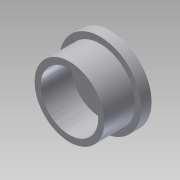
# Autodesk Inventor part: Bouchon PVC
Saved by Autodesk Inventor 2016 (Build 200138000, 138)
## iProperties
Created: 2016-01-27
Part Number: Bouchon PVC
Material: PVC, non plastifié
Document SubType Name: Modeling
Designer: sd
Mass: 14.2475 g
Surface Area: 61.3475 cm^2
Volume: 10.1768 cm^3
Density: 1.4 g/cm^3
Appearance: Lisse - Blanc
Author: sd
Autodesk Inventor part; units mm, degrees
ref_plane "YZ Plane" through (0, 0, 0) normal (1, 0, 0) x (0, 1, 0)
ref_plane "XZ Plane" through (0, 0, 0) normal (0, 1, 0) x (-1, 0, 0)
ref_plane "XY Plane" through (0, 0, 0) normal (0, 0, 1) x (1, 0, 0)
sketch "Esquisse1" plane through (0, 0, 0) normal (0, 1, 0) x (-1, 0, 0)
  circle A0 centre (0, 0) radius 20
  dimension "d0" = 40
  constraints: 1 centre point, 1 coincident
  measures "d0" diameter of A0
extrude "Extrusion1" add sketch "Esquisse1" along normal blind 20
sketch "Esquisse2" plane through (0, 0, 0) normal (0, -1, 0) x (1, 0, 0)
  circle A0 centre (0, 0) radius 20 projected
  circle A1 centre (0, 0) radius 17
  dimension "d3" = 3
  constraints: 1 centre point, 1 coincident
  measures "d3" radial gap between concentric circles of A0 A1
extrude "Extrusion2" cut sketch "Esquisse2" against normal blind 15
sketch "Esquisse3" plane through (0, 0, 0) normal (0, -1, 0) x (1, 0, 0)
  circle A0 centre (0, 0) radius 17 projected
  circle A1 centre (0, 0) radius 14
  dimension "d6" = 3
  constraints: 1 centre point, 1 coincident
  measures "d6" radial gap between concentric circles of A0 A1
extrude "Extrusion3" cut sketch "Esquisse3" against normal blind 15 contours A1
sketch "Esquisse4" plane through (0, 15, 0) normal (0, -1, 0) x (1, 0, 0)
  circle A0 centre (0, 0) radius 14 projected
  circle A1 centre (0, 0) radius 5
  circle A2 centre (0, 11) radius 1.75
  circle A3 centre (0, -11) radius 1.75
  dimension "d9" = 10
  dimension "d10" = 3.5
  dimension "d11" = 3.5
  dimension "d12" = 11
  dimension "d13" = 11
  constraints: 3 centre point, 1 coincident
  measures "d9" diameter of A1
  measures "d10" diameter of A2
  measures "d11" diameter of A3
  measures "d12" distance of A0.centre A3.centre
  measures "d13" distance of A0.centre A2.centre
extrude "Extrusion4" cut sketch "Esquisse4" against normal through all contours A1 | A2 | A3
equation "\"d11\" = d10"
equation "\"d13\" = d12"
